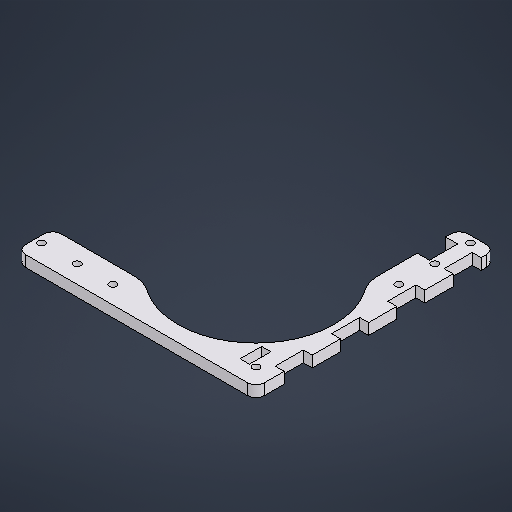
# Autodesk Inventor part: INTAKE_SWERVE_MOUNT
Saved by Autodesk Inventor 2026 (Build 300175000, 175)
## iProperties
Created: 2026-04-01
Part Number: INTAKE_SWERVE_MOUNT
Material: Aluminum, 6061-T6
Document SubType Name: Sheet Metal
Designer: 4aida
Density: 2.71 g/cm^3
Sheet Metal Rule: Default_mm
Appearance: Metal-AL-6061 (Flat)
Author: 4aida
Autodesk Inventor part; units mm, degrees
ref_plane "YZ Plane" through (0, 0, 0) normal (1, 0, 0) x (0, 1, 0)
ref_plane "XZ Plane" through (0, 0, 0) normal (0, 1, 0) x (-1, 0, 0)
ref_plane "XY Plane" through (0, 0, 0) normal (0, 0, 1) x (1, 0, 0)
sketch "Sketch1" plane through (0, 0, 0) normal (0, 1, 0) x (-1, 0, 0)
  line L0 (169.8625, 0) -> (0, 0)
  line L1 (0, 0) -> (0, -169.8625)
  line L2 (0, -169.8625) -> (25.4, -169.8625)
  line L3 (25.4, -169.8625) -> (25.4, -103.8713)
  line L4 (103.8713, -25.4) -> (169.8625, -25.4)
  line L5 (169.8625, -25.4) -> (169.8625, 0)
  arc A0 (103.8713, -25.4) -> (25.4, -103.8713) centre (66.675, -66.675) ccw
  line L6 (0, 0) -> (66.675, -66.675) construction
  line L7 (0, -20) -> (6.35, -20)
  line L8 (6.35, -20) -> (6.35, -40)
  line L9 (6.35, -40) -> (0, -40)
  line L10 (0, -40) -> (0, -20)
  line L11 (6.35, -60) -> (6.35, -80)
  line L12 (0, -60) -> (6.35, -60)
  line L13 (6.35, -80) -> (0, -80)
  line L14 (6.35, -100) -> (6.35, -120)
  line L15 (0, -100) -> (6.35, -100)
  line L16 (6.35, -120) -> (0, -120)
  line L17 (6.35, -140) -> (6.35, -160)
  line L18 (0, -140) -> (6.35, -140)
  line L19 (6.35, -160) -> (0, -160)
  line L20 (23.368, -27.3469) -> (16.764, -27.3469)
  line L21 (16.764, -27.3469) -> (16.764, -12.0929)
  line L22 (16.764, -12.0929) -> (23.368, -12.0929)
  line L23 (23.368, -12.0929) -> (23.368, -27.3469)
  line L24 (23.368, -27.3469) -> (16.764, -12.0929) construction
  line L25 (16.764, -27.3469) -> (23.368, -12.0929) construction
  line L26 (25.4, -160) -> (16.764, -160)
  line L27 (16.764, -160) -> (16.764, -140)
  line L28 (16.764, -140) -> (25.4, -140)
  point P0 (103.8713, -25.4)
  point P1 (20.066, -19.7199)
  point P2 (20.066, -12.0929)
  dimension "d0" = 25.4
  dimension "d1" = 169.8625
  dimension "d2" = 25.4
  dimension "d3" = 169.8625
  dimension "d4" = 111.125
  dimension "d5" = 66.675
  dimension "d6" = 45
  dimension "d10" = 6.35
  dimension "d11" = 20
  dimension "d12" = 20
  dimension "d15" = 40
  dimension "d34" = 12.0929
  dimension "d35" = 6.604
  dimension "d36" = 20.066
  dimension "d37" = 15.254
  measures "d0" distance between parallel lines of L4 L0
  measures "d1" distance between parallel lines of L1 L5
  measures "d2" distance of L1.end L2.end
  measures "d3" distance between parallel lines of L0 L2
  measures "d4" diameter of A0
  measures "d5" distance from line of L1 L6.end
  measures "d6" angle of L1 L6
  measures "d10" distance between parallel lines of L1 L8
  measures "d11" distance of L7.end L8.end
  measures "d12" distance between parallel lines of L7 L0
  measures "d15" distance of L7.end L11.start
  measures "d34" distance between parallel lines of L0 L22
  measures "d35" distance of L21.end L22.end
  measures "d36" distance from line of L1 point (20.066, -12.093)
  measures "d37" distance of L22.end L20.start
extrude "Plate1" add sketch "Sketch1" along normal blind 7.9375 contours L5 L4 A0 L3 L28 L27 L26 L2 L1 L19 L17 L18 L16 L14 L15 L13 L11 L12 L9 L8 L7 L0
fillet "Corner Round1" radius 25.4 2 edges at (-103.8713, 3.9688, -25.4) (-25.4, 3.9688, -103.8713)
fillet "Corner Round2" radius 6 5 edges at (0, 3.9688, 0) (0, 3.9688, -169.8625) (-25.4, 3.9688, -169.8625) (-169.8625, 3.9688, 0) (-169.8625, 3.9688, -25.4)
sketch "Sketch2" plane through (0, 0, 0) normal (0, -1, 0) x (1, 0, 0)
  line L0 (-169.8625, -19.4) -> (-169.8625, -6) projected
  line L1 (-19.4, -169.8625) -> (-6, -169.8625) projected
  line L2 (-6, -169.8625) -> (-19.4, -169.8625) projected
  line L3 (0, -20) -> (0, -6) projected
  line L4 (-6, 0) -> (-163.8625, 0) projected
  point P0 (0, 0)
  point P1 (-165.1, -12.7)
  point P2 (-139.7, -12.7)
  point P3 (-114.3, -12.7)
  point P4 (-12.7, -165.1)
  point P5 (-12.7, -139.7)
  point P6 (-12.7, -114.3)
  point P7 (-169.8625, -12.7)
  point P8 (-169.8625, -12.7)
  point P9 (-12.7, -169.8625)
  point P10 (-12.7, -12.7)
  dimension "d21" = 25.4
  dimension "d22" = 25.4
  dimension "d23" = 25.4
  dimension "d24" = 25.4
  dimension "d25" = 4.7625
  dimension "d26" = 4.7625
  dimension "d38" = 12.7
  dimension "d39" = 12.7
  constraints: 3 horizontal alignment, 3 midpoint, 3 vertical alignment
  measures "d21" distance of point (-139.7, -12.7) point (-114.3, -12.7)
  measures "d22" distance of point (-165.1, -12.7) point (-139.7, -12.7)
  measures "d23" distance of point (-12.7, -139.7) point (-12.7, -165.1)
  measures "d24" distance of point (-12.7, -139.7) point (-12.7, -114.3)
  measures "d25" distance of point (-169.863, -12.7) point (-165.1, -12.7)
  measures "d26" distance from line of L1 point (-12.7, -165.1)
  measures "d38" distance from line of L3 point (-12.7, -12.7)
  measures "d39" distance from line of L4 point (-12.7, -12.7)
hole "Hole1" at (-165.1, 0, -12.7) at (-139.7, 0, -12.7) at (-114.3, 0, -12.7) at (-12.7, 0, -165.1) at (-12.7, 0, -139.7) at (-12.7, 0, -114.3) at (-12.7, 0, -12.7) direction (0, 1, 0) diameter 5.105 depth 7.9375 tip angle 118 clearance for "Flat Head Machine Screw (82)" size "#10" standard "Ansi Unified Screw Threads"
equation "\"d22\" = d21"
equation "\"d23\" = d21"
equation "\"d24\" = d23"
equation "\"d2\" = d0"
equation "\"d3\" = d1"
equation "\"d12\" = d11"
equation "\"d15\" = 2 * d11"
equation "\"d32\" = Thickness"
equation "\"d8\" = Thickness"
equation "\"BendRadius\" = Thickness"
equation "\"BendReliefWidth\" = Thickness"
equation "\"BendReliefDepth\" = 0.5 * Thickness"
equation "\"CornerReliefSize\" = 4 * Thickness"
equation "\"MinimumRemnant\" = 2 * Thickness"
equation "\"TransitionRadius\" = BendRadius"
equation "\"JacobiRadiusSize\" = BendRadius"
equation "\"GapSize\" = Thickness"
equation "\"Thickness\" = 7.9375"
body "Solid1"
